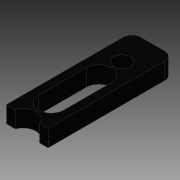
# Autodesk Inventor part: Fixture_Slide_Lock_Plate
Saved by Autodesk Inventor 2015 (Build 190159000, 159)
## iProperties
Created: 2014-12-16
Part Number: Fixture_Slide_Lock_Plate
Material: Generic
Document SubType Name: Modeling
Designer: amarschn
Density: 1 g/cm^3
Appearance: Anodized - Black
Author: amarschn
Autodesk Inventor part; units mm, degrees
ref_plane "YZ Plane" through (0, 0, 0) normal (1, 0, 0) x (0, 1, 0)
ref_plane "XZ Plane" through (0, 0, 0) normal (0, 1, 0) x (-1, 0, 0)
ref_plane "XY Plane" through (0, 0, 0) normal (0, 0, 1) x (1, 0, 0)
sketch "Sketch1" plane through (0, 0, 0) normal (0, 1, 0) x (-1, 0, 0)
  line L0 (-9.2075, -46.99) -> (9.2075, -46.99)
  line L1 (15.5575, -40.64) -> (15.5575, 46.99)
  line L2 (-15.5575, 46.99) -> (-15.5575, -40.64)
  line L3 (-15.5575, -46.99) -> (15.5575, 46.99) construction
  line L4 (15.5575, -46.99) -> (-15.5575, 46.99) construction
  circle A0 centre (0, -24.13) radius 6.35
  line L5 (9.525, -6.6675) -> (9.525, 29.21)
  line L6 (-9.525, 29.21) -> (-9.525, -6.6675)
  line L7 (-9.525, -6.6675) -> (9.525, 29.21) construction
  line L8 (9.525, -6.6675) -> (-9.525, 29.21) construction
  arc A1 (9.525, 29.21) -> (-9.525, 29.21) centre (0, 29.21) ccw
  arc A2 (-9.525, -6.6675) -> (9.525, -6.6675) centre (0, -6.6675) ccw
  line L9 (-8.89, 46.99) -> (-15.5575, 46.99)
  arc A3 (9.2075, -46.99) -> (15.5575, -40.64) centre (9.2075, -40.64) ccw
  arc A4 (-15.5575, -40.64) -> (-9.2075, -46.99) centre (-9.2075, -40.64) ccw
  line L10 (0, 71.5612) -> (0, -73.6541)
  arc A5 (-8.9803, 46.99) -> (8.9803, 46.99) centre (0, 50.165) ccw
  line L11 (15.5575, 46.99) -> (8.9803, 46.99)
  line L12 (-8.9803, 46.99) -> (-15.5575, 46.99)
  point P0 (0, 0)
  point P1 (0, 11.2712)
  point P2 (0, 0)
  point P3 (0, 11.2712)
  dimension "d0" = 93.98
  dimension "d1" = 31.115
  dimension "d2" = 22.86
  dimension "d3" = 12.7
  dimension "d4" = 35.8775
  dimension "d5" = 19.05
  dimension "d7" = 6.35
  dimension "d12" = 19.05
  dimension "d13" = 17.78
  dimension "d14" = 3.175
  constraints: 26 end point, 10 point on circle, 10 point on line, 8 tangent, 6 centre point, 6 midpoint, 5 parallel, 2 collinear, 1 equal radius, 1 horizontal, 1 perpendicular, 1 vertical
  measures "d0" distance of L4.start L1.end
  measures "d1" distance of L3.start L4.start
  measures "d2" distance from line of L0 A0.centre
  measures "d3" diameter of A0
  measures "d4" distance of A2.centre A1.centre
  measures "d5" distance between parallel lines of L6 L5
  measures "d7" radius of A3
  measures "d12" diameter of A5
  measures "d13" distance from line of L9 A1.centre
  measures "d14" distance from line of L12 A5.centre
extrude "Extrusion1" add sketch "Sketch1" along normal blind 12.7 contours A4 L2 L9 A5 L10 A1 L6 A2 A0 L0 | L10 A0 A2 L5 A1 A5 L11 L1 A3 L0
equation "\"d12\" = d5"
body "Solid1"
